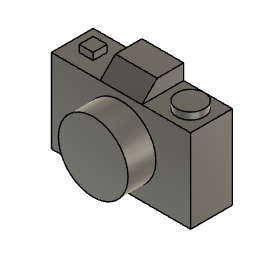
camera v1 (Autodesk Fusion 360 design; units mm, degrees)
Autodesk Fusion 360 part; units mm, degrees
sketch "Sketch1" plane through (0, 0, 0) normal (0, 1, 0) x (1, 0, 0)
  line L0 (50, 30) -> (-50, 30)
  line L1 (-50, 30) -> (-50, -30)
  line L2 (-50, -30) -> (50, -30)
  line L3 (50, -30) -> (50, 30)
  line L4 (50, 30) -> (-50, -30) construction
  line L5 (-50, 30) -> (50, -30) construction
  dimension "d1" = 100
  dimension "d2" = 60
  constraint horizontal L0
  constraint perpendicular L0 L1
  constraint parallel L0 L2
  constraint parallel L1 L3
  constraint coincident L4 origin
  constraint coincident L5 origin
  measures "d1" distance of L1.end L2.end
  measures "d2" distance of L0.end L1.end
extrude "Extrude1" add sketch "Sketch1" along normal blind 30
sketch "Sketch2" plane through (0, 0, 0) normal (0, -1, 0) x (1, 0, 0)
  line L0 (50, -30) -> (50, 30)
  line L1 (50, 30) -> (-50, 30)
  line L2 (-50, 30) -> (-50, -30)
  line L3 (-50, -30) -> (50, -30)
  circle A0 centre (0, 0) radius 25
  dimension "d5" = 50
  constraint coincident A0.centre origin
  measures "d5" diameter of A0
extrude "Extrude2" add sketch "Sketch2" along normal blind 20 contours A0
sketch "Sketch3" plane through (0, 0, 30) normal (0, 0, 1) x (-1, 0, 0)
  line L0 (50, 0) -> (-50, 0)
  line L1 (-50, 0) -> (-50, -30)
  line L2 (-50, -30) -> (50, -30)
  line L3 (50, -30) -> (50, 0)
  circle A0 centre (-35, -15) radius 10
  dimension "d8" = 20
  dimension "d9" = 15
  dimension "d10" = 15
  measures "d8" diameter of A0
  measures "d9" distance of L2 A0.centre
  measures "d10" distance of L1 A0.centre
extrude "Extrude3" add sketch "Sketch3" along normal blind 5 contours A0
sketch "Sketch4" plane through (0, 0, 30) normal (0, 0, 1) x (-1, 0, 0)
  circle A0 centre (-35, -15) radius 10
  line L0 (50, 0) -> (-50, 0)
  line L1 (-50, 0) -> (-50, -30)
  line L2 (-50, -30) -> (50, -30)
  line L3 (50, -30) -> (50, 0)
  line L4 (30, -10) -> (40, -10)
  line L5 (40, -10) -> (40, -20)
  line L6 (40, -20) -> (30, -20)
  line L7 (30, -20) -> (30, -10)
  line L8 (30, -10) -> (40, -20) construction
  line L9 (40, -10) -> (30, -20) construction
  point P0 (35, -15)
  dimension "d13" = 10
  dimension "d14" = 10
  dimension "d15" = 15
  dimension "d16" = 15
  constraint horizontal L4
  constraint perpendicular L4 L5
  constraint parallel L4 L6
  constraint parallel L5 L7
  constraint coincident L8 P0
  constraint coincident L9 P0
  measures "d13" distance of L5.end L6.end
  measures "d14" distance of L4.end L5.end
  measures "d15" distance of L2 P0
  measures "d16" distance of L3 P0
extrude "Extrude4" add sketch "Sketch4" along normal blind 5 contours L4 L5 L6 L7
box "BoxPrimitive1" add length 30 width 30 height 1 placed x (0, -1, 0) y (1, 0, 0) z (0, 0, 1) at (-15, 30, 30)
extrude "Extrude5" add 1 faces at (-5, 10, 31) along direction (0, 0, 1) blind 10
sketch "Sketch6" plane through (15, 0, 0) normal (1, 0, 0) x (0, 1, 0)
  line L0 (0, 41) -> (0, 30)
  line L1 (0, 30) -> (30, 30)
  line L2 (30, 30) -> (30, 41)
  line L3 (30, 41) -> (0, 41)
  line L4 (0, 30) -> (11, 41)
  line L5 (0, 30) -> (15.5563, 30) construction
  dimension "d26" = 45
  constraint horizontal L5
  constraint coincident L0.end L1.start
  constraint coincident L3 L4.end
  measures "d26" angle of L4 L5
extrude "Extrude6" cut sketch "Sketch6" against normal blind 30 contours L0 L3 L4
